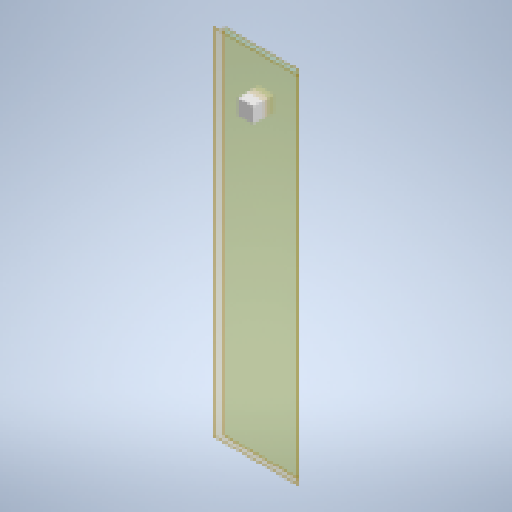
# Autodesk Inventor part: Camera
Saved by Autodesk Inventor 2027.1 (Build 311270010, 270A)
## iProperties
Created: 2026-09-10
Part Number: Camera
Material: Generic
Document SubType Name: Modeling
Designer: PWYNNE
Density: 1 g/cm^3
Appearance: Default
Author: PWYNNE
Autodesk Inventor part; units mm, degrees
ref_plane "YZ Plane" through (0, 0, 0) normal (1, 0, 0) x (0, 1, 0)
ref_plane "XZ Plane" through (0, 0, 0) normal (0, 1, 0) x (-1, 0, 0)
ref_plane "XY Plane" through (0, 0, 0) normal (0, 0, 1) x (1, 0, 0)
ref_plane "Work Plane1" through (0, 0, -10) normal (0, 0, -1) x (-1, 0, 0)
ref_plane "Work Plane2" through (0, 0, 0) normal (0, 0, 1) x (1, 0, 0)
sketch "Sketch1" plane through (0, 0, 0) normal (0, 0, 1) x (1, 0, 0)
  line L0 (15, 360) -> (135, 360) projected
  line L1 (0, -150) -> (150, -150) projected
  line L2 (150, -150) -> (150, 350) projected
  spline S0 degree 4 poles (150, 350) (150, 390.8194) (138.5388, 426.4442) (123.0072, 457.9209) (107.5607, 478.2829) knots -2 -2 -2 -2 -2 -1.381907 -1.381907 -1.381907 -1.381907 -1.381907 projected
  line L3 (42.4393, 478.2829) -> (107.5607, 478.2829) projected
  spline S1 degree 4 poles (42.4393, 478.2829) (26.9928, 457.9209) (11.4612, 426.4442) (0, 390.8194) (0, 350) knots -1.618093 -1.618093 -1.618093 -1.618093 -1.618093 -1 -1 -1 -1 -1 projected
  line L4 (0, -150) -> (0, 350) projected
  line L5 (75, 478.2829) -> (75, 360)
  line L6 (60, 404.1414) -> (90, 404.1414)
  line L7 (90, 404.1414) -> (90, 434.1414)
  line L8 (90, 434.1414) -> (60, 434.1414)
  line L9 (60, 434.1414) -> (60, 404.1414)
  line L10 (60, 404.1414) -> (90, 434.1414) construction
  line L11 (90, 404.1414) -> (60, 434.1414) construction
  point P0 (0, 0)
  point P1 (75, 419.1414)
  dimension "d0" = 30
  dimension "d1" = 30
  constraints: 14 end point, 5 midpoint, 2 parallel, 1 horizontal, 1 perpendicular
  measures "d0" distance of L8.end L7.end
  measures "d1" distance of L7.end L6.end
extrude "Extrusion1" add sketch "Sketch1" along normal mid plane 50 contours L8 L7 L6 L5 | L5 L6 L9 L8
body "Solid1"
